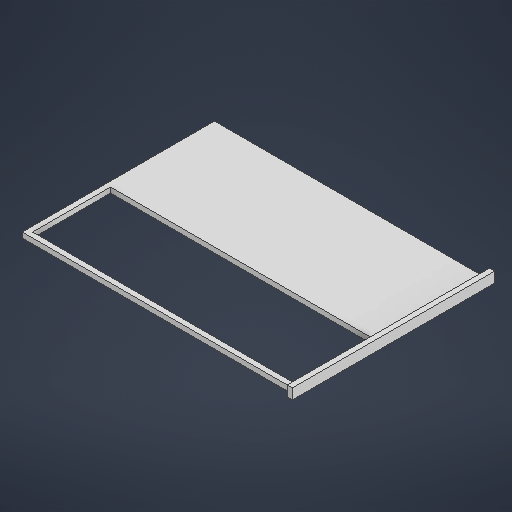
# Autodesk Inventor part: Lid
Saved by Autodesk Inventor 2027.1 (Build 311270010, 270A)
## iProperties
Created: 2026-10-08
Part Number: Lid
Material: Generic
Document SubType Name: Modeling
Designer: Richard
Density: 1 g/cm^3
Appearance: Default
Author: Richard
Autodesk Inventor part; units mm, degrees
ref_plane "YZ Plane" through (0, 0, 0) normal (1, 0, 0) x (0, 1, 0)
ref_plane "XZ Plane" through (0, 0, 0) normal (0, 1, 0) x (-1, 0, 0)
ref_plane "XY Plane" through (0, 0, 0) normal (0, 0, 1) x (1, 0, 0)
sketch "Sketch1" plane through (0, 0, 0) normal (0, 1, 0) x (-1, 0, 0)
  line L0 (0, 0) -> (-104, 0)
  line L1 (-104, 0) -> (-104, -74)
  line L2 (-104, -74) -> (0, -74)
  line L3 (0, -74) -> (0, 0)
  line L4 (-104, 2) -> (-106, 2)
  line L5 (-106, 2) -> (-106, -76)
  line L6 (-106, -76) -> (-104, -76)
  line L7 (-104, -76) -> (-104, 2)
  line L8 (-2, -2) -> (-102, -2)
  line L9 (-102, -2) -> (-102, -32)
  line L10 (-102, -32) -> (-2, -32)
  line L11 (-2, -32) -> (-2, -2)
  dimension "d0" = 104
  dimension "d1" = 74
  dimension "d2" = 2
  dimension "d3" = 78
  dimension "d4" = 104
  dimension "d5" = 2
  dimension "d6" = 100
  dimension "d7" = 30
  dimension "d8" = 2
  dimension "d9" = 2
  constraints: 24 end point, 6 parallel, 3 horizontal, 3 perpendicular
  measures "d0" distance of L2.end L1.end
  measures "d1" distance of L1.end L0.end
  measures "d2" distance of L6.end L5.end
  measures "d3" distance of L5.end L4.end
  measures "d4" distance between parallel lines of L7 L3
  measures "d5" distance between parallel lines of L4 L0
  measures "d6" distance of L10.end L9.end
  measures "d7" distance of L9.end L8.end
  measures "d8" distance between parallel lines of L11 L3
  measures "d9" distance between parallel lines of L8 L0
extrude "Extrusion1" add sketch "Sketch1" along normal blind 4 contours L1 L7 L6 L5 L4
extrude "Extrusion2" add sketch "Sketch1" along normal blind 2 contours L3 L2 L1 L0
body "Solid1"
